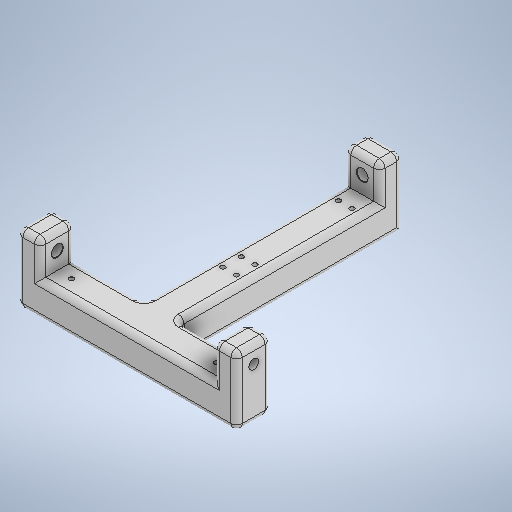
# Autodesk Inventor part: Tcalev2
Saved by Autodesk Inventor 2025.3 (Build 293356000, 356)
## iProperties
Created: 2026-05-17
Part Number: Tcalev2
Material: Generic
Document SubType Name: Modeling
Designer: ksawe
Density: 1 g/cm^3
Appearance: Default
Author: ksawe
Autodesk Inventor part; units mm, degrees
ref_plane "YZ Plane" through (0, 0, 0) normal (1, 0, 0) x (0, 1, 0)
ref_plane "XZ Plane" through (0, 0, 0) normal (0, 1, 0) x (-1, 0, 0)
ref_plane "XY Plane" through (0, 0, 0) normal (0, 0, 1) x (1, 0, 0)
sketch "Sketch1" plane through (0, 0, 0) normal (0, 1, 0) x (-1, 0, 0)
  line L0 (96, 15) -> (-96, 15)
  line L1 (-96, 15) -> (-96, -15)
  line L2 (96, -15) -> (96, 15)
  line L3 (96, 15) -> (-96, -15) construction
  line L4 (-96, 15) -> (96, -15) construction
  line L5 (0, 0) -> (0, -223) construction
  line L6 (15, -211.066) -> (15, -15)
  line L7 (-96, -15) -> (-15, -15)
  line L8 (15, -15) -> (96, -15)
  line L9 (-15, -211.066) -> (-15, -15)
  line L10 (15, -211.066) -> (-15, -211.066)
  dimension "d0" = 192
  dimension "d1" = 30
  dimension "d2" = 196.066
  dimension "d3" = 15
  constraints: 22 end point, 3 parallel, 3 perpendicular, 2 horizontal, 2 midpoint, 2 symmetric about line, 1 vertical
  measures "d0" distance of L0.start L0.end
  measures "d1" distance of L0.end L1.end
  measures "d2" distance of L6.start L6.end
  measures "d3" distance between parallel lines of L5 L6
extrude "Extrusion1" add sketch "Sketch1" along normal mid plane 30
sketch "Sketch2" plane through (0, 15, 0) normal (0, 1, 0) x (1, 0, 0)
  line L0 (15, 15) -> (96, 15) projected
  line L1 (96, -15) -> (-96, -15) projected
  line L2 (96, 15) -> (76, 15)
  line L3 (76, 15) -> (76, -15)
  line L4 (76, -15) -> (96, -15)
  line L5 (96, -15) -> (96, 15)
  line L6 (15, 211.066) -> (15, 15) projected
  line L7 (-15, 15) -> (-15, 211.066) projected
  line L8 (15, 211.066) -> (-15, 211.066)
  line L9 (-15, 211.066) -> (-15, 191.066)
  line L10 (-15, 191.066) -> (15, 191.066)
  line L11 (15, 191.066) -> (15, 211.066)
  line L12 (-96, 15) -> (-15, 15) projected
  line L13 (-96, -15) -> (-76, -15)
  line L14 (-76, -15) -> (-76, 15)
  line L15 (-76, 15) -> (-96, 15)
  line L16 (-96, 15) -> (-96, -15)
  point P0 (0, 0)
  point P1 (-15, 211.066)
  point P2 (15, 191.066)
  point P3 (76, 15)
  point P4 (-76, -15)
  dimension "d6" = 20
  dimension "d7" = 20
  dimension "d8" = 20
  constraints: 24 end point, 6 parallel, 3 horizontal, 3 perpendicular, 3 point on line
  measures "d6" distance between parallel lines of L8 L10
  measures "d7" distance between parallel lines of L5 L3
  measures "d8" distance between parallel lines of L14 L16
extrude "Extrusion2" add sketch "Sketch2" along normal blind 30 contours L0 L5 L1 L3 | L10 L7 L8 L6 | L1 L16 L12 L14
fillet "Fillet1" radius 5 38 edges at (15, 0, -15) (-15, 0, -15) (15, -15, -113.033) (55.5, -15, -15) (-55.5, -15, -15) (0, -15, 15) (96, -15, 0) (96, 15, -15) (96, 15, 15) (96, 45, 0) (-96, 15, 15) (-96, -15, 0) (-96, 15, -15) (-96, 45, 0) (-15, 15, -211.066) (15, 15, -211.066) (0, 45, -211.066) (0, 45, -191.066) (0, 15, 15) (-76, 45, 0) (-86, 45, 15) (-86, 45, -15) (86, 45, -15) (86, 45, 15) (76, 45, 0) (15, 45, -201.066) (-15, 45, -201.066) (76, 30, 15) (76, 30, -15) (-76, 30, 15) (-76, 30, -15) (15, 30, -191.066) (-15, 30, -191.066) (-15, -15, -113.033) (-15, 15, -103.033) (15, 15, -103.033) (45.5, 15, -15) (-45.5, 15, -15)
sketch "Sketch3" plane through (0, 15, 0) normal (0, 1, 0) x (1, 0, 0)
  line L0 (-76, 10) -> (-76, -10) projected
  line L1 (-81, -15) -> (81, -15) projected
  line L2 (76, -10) -> (76, 10) projected
  line L3 (-15, 196.066) -> (-15, 20) projected
  line L4 (-10, 191.066) -> (10, 191.066) projected
  line L5 (10, 191.066) -> (-10, 191.066) projected
  line L6 (15, 20) -> (15, 196.066) projected
  point P0 (0, 0)
  point P1 (-63.5, 0)
  point P2 (63.5, 0)
  point P3 (6, 176.066)
  point P4 (-6, 176.066)
  point P5 (6, 91.066)
  point P6 (-6, 91.066)
  point P7 (-6, 75)
  point P8 (6, 75)
  dimension "d19" = 12.5
  dimension "d20" = 15
  dimension "d21" = 15
  dimension "d22" = 12.5
  dimension "d23" = 90
  dimension "d24" = 90
  dimension "d25" = 9
  dimension "d26" = 100
  dimension "d27" = 9
  dimension "d28" = 100
  dimension "d29" = 9
  dimension "d30" = 9
  dimension "d58" = 15
  dimension "d59" = 15
  dimension "d60" = 9
  dimension "d61" = 9
  measures "d19" distance from line of L0 point (-63.5, 0)
  measures "d20" distance from line of L1 point (-63.5, 0)
  measures "d21" distance from line of L1 point (63.5, 0)
  measures "d22" distance from line of L2 point (63.5, 0)
  measures "d23" distance from line of L1 point (6, 75)
  measures "d24" distance from line of L1 point (-6, 75)
  measures "d25" distance from line of L3 point (-6, 75)
  measures "d26" distance from line of L4 point (-6, 91.066)
  measures "d27" distance from line of L3 point (-6, 91.066)
  measures "d28" distance from line of L5 point (6, 91.066)
  measures "d29" distance from line of L6 point (6, 91.066)
  measures "d30" distance from line of L6 point (6, 75)
  measures "d58" distance from line of L5 point (6, 176.066)
  measures "d59" distance from line of L5 point (-6, 176.066)
  measures "d60" distance from line of L6 point (6, 176.066)
  measures "d61" distance from line of L3 point (-6, 176.066)
hole "Hole1" at (-63.5, 15, 0) at (63.5, 15, 0) at (-6, 15, -91.066) at (6, 15, -91.066) at (6, 15, -75) at (-6, 15, -75) at (6, 15, -176.066) at (-6, 15, -176.066) direction (0, -1, 0) diameter 4 depth 7 countersink diameter 4.2 countersink angle 90
sketch "Sketch7" plane through (76, 15, -10) normal (-1, 0, 0) x (0, 0, 1)
  line L0 (-5, 25) -> (-5, -5) projected
  line L1 (20, 30) -> (0, 30) projected
  point P0 (10, -15)
  point P1 (10, 15)
  dimension "d83" = 15
  dimension "d84" = 15
  measures "d83" distance from line of L0 point (10, 15)
  measures "d84" distance from line of L1 point (10, 15)
hole "Hole5" at (76, 30, 0) direction (1, 0, 0) diameter 9.8 depth 10.5 countersink diameter 10.5 countersink angle 90
sketch "Sketch8" plane through (-76, 15, 10) normal (1, 0, 0) x (0, 0, -1)
  line L0 (20, 30) -> (0, 30) projected
  line L1 (25, -5) -> (25, 25) projected
  point P0 (10, -15)
  point P1 (10, 15)
  dimension "d85" = 15
  dimension "d86" = 15
  measures "d85" distance from line of L0 point (10, 15)
  measures "d86" distance from line of L1 point (10, 15)
hole "Hole6" at (-76, 30, 0) direction (-1, 0, 0) diameter 9.8 depth 10.5 countersink diameter 10.5 countersink angle 90
sketch "Sketch9" plane through (-10, 15, -191.066) normal (0, 0, 1) x (1, 0, 0)
  line L0 (-5, 25) -> (-5, -5) projected
  line L1 (20, 30) -> (0, 30) projected
  point P0 (10, -15)
  point P1 (10, 15)
  dimension "d87" = 15
  dimension "d88" = 15
  measures "d87" distance from line of L0 point (10, 15)
  measures "d88" distance from line of L1 point (10, 15)
hole "Hole7" at (0, 30, -191.066) direction (0, 0, -1) diameter 9.8 depth 10.5 countersink diameter 10.5 countersink angle 90
sketch "Sketch10" plane through (96, -10, -10) normal (1, 0, 0) x (0, 0, -1)
  line L0 (0, 55) -> (-20, 55) projected
  line L1 (5, 0) -> (5, 50) projected
  point P0 (-10, 10)
  point P1 (-10, 40)
  dimension "d89" = 15
  dimension "d90" = 15
  measures "d89" distance from line of L0 point (-10, 40)
  measures "d90" distance from line of L1 point (-10, 40)
hole "Hole8" at (96, 30, 0) direction (-1, 0, 0) diameter 8.5 end through all
sketch "Sketch11" plane through (10, 40, -211.066) normal (0, 0, -1) x (-1, 0, 0)
  line L0 (20, 5) -> (0, 5) projected
  line L1 (25, -50) -> (25, 0) projected
  point P0 (10, -40)
  point P1 (10, -10)
  dimension "d98" = 15
  dimension "d99" = 15
  measures "d98" distance from line of L0 point (10, -10)
  measures "d99" distance from line of L1 point (10, -10)
hole "Hole9" at (0, 30, -211.066) direction (0, 0, 1) diameter 8.5 end through all
body "Solid1"
